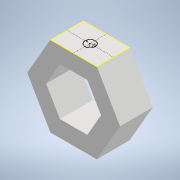
# Autodesk Inventor part: Hombro_Ejes
Saved by Autodesk Inventor 2022 (Build 260153000, 153)
## iProperties
Created: 2022-02-21
Part Number: Hombro_Ejes
Material: Generic
Document SubType Name: Modeling
Designer: katha
Density: 1 g/cm^3
Appearance: Default
Author: katha
Autodesk Inventor part; units mm, degrees
ref_plane "YZ Plane" through (0, 0, 0) normal (1, 0, 0) x (0, 1, 0)
ref_plane "XZ Plane" through (0, 0, 0) normal (0, 1, 0) x (-1, 0, 0)
ref_plane "XY Plane" through (0, 0, 0) normal (0, 0, 1) x (1, 0, 0)
sketch "Sketch1" plane through (0, 0, 0) normal (0, 0, 1) x (1, 0, 0)
  line L0 (1.6732, 2.8981) -> (-1.6732, 2.8981) projected
  line L1 (-1.6732, 2.8981) -> (-3.3464, 0) projected
  line L2 (-3.3464, 0) -> (-1.6732, -2.8981) projected
  line L3 (-1.6732, -2.8981) -> (1.6732, -2.8981) projected
  line L4 (1.6732, -2.8981) -> (3.3464, 0) projected
  line L5 (3.3464, 0) -> (1.6732, 2.8981) projected
  line L6 (-2.8279, 4.8981) -> (2.8279, 4.8981)
  line L7 (2.8279, 4.8981) -> (5.6558, 0)
  line L8 (5.6558, 0) -> (2.8279, -4.8981)
  line L9 (2.8279, -4.8981) -> (-2.8279, -4.8981)
  line L10 (-2.8279, -4.8981) -> (-5.6558, 0)
  line L11 (-5.6558, 0) -> (-2.8279, 4.8981)
  point P0 (0, 0)
  dimension "d0" = 2
  constraints: 12 end point, 5 other
  measures "d0" distance between parallel lines of L0 L6
extrude "Extrusion1" add sketch "Sketch1" along normal blind 5
sketch "Sketch2" plane through (-2.8279, 4.8981, 0) normal (0, 1, 0) x (1, 0, 0)
  line L0 (0, 0) -> (0, -5) projected
  line L1 (5.6558, -5) -> (0, -5) projected
  line L2 (5.6558, 0) -> (5.6558, -5) projected
  line L3 (5.6558, 0) -> (0, 0) projected
  line L4 (0, 0) -> (0, -5) projected
  line L5 (0, -2.5) -> (5.6558, -2.5) construction
  line L6 (5.6558, 0) -> (5.6558, -5) projected
  line L7 (4.5011, -5) -> (1.1547, -5) projected
  line L8 (2.8279, -5) -> (2.8279, 0) construction
  circle A0 centre (2.8279, -2.5) radius 0.625
  dimension "d3" = 1.25
  constraints: 4 end point, 4 midpoint, 1 centre point, 1 perpendicular
  measures "d3" diameter of A0
extrude "Extrusion2" cut sketch "Sketch2" against normal blind 10 contours A0
body "Solid1"
